Autodesk Inventor part; units mm, degrees
(part 2 of 5)
  arc A560 (53.3588, 33.4823) -> (53.3762, 34.0151) centre (44.1675, 34.0494) ccw
  arc A561 (53.3762, 34.0151) -> (53.35, 34.4073) centre (50.5813, 34.0255) ccw
  arc A562 (53.35, 34.4073) -> (53.2888, 34.6516) centre (52.1975, 34.2484) ccw
  arc A563 (53.2888, 34.6516) -> (53.1912, 34.6976) centre (53.2166, 34.6249) ccw
  arc A564 (53.1912, 34.6976) -> (53.0949, 34.5943) centre (53.2411, 34.5546) ccw
  arc A565 (53.0949, 34.5943) -> (53.0197, 34.2521) centre (56.5471, 33.6564) ccw
  arc A566 (53.0197, 34.2521) -> (52.9689, 33.8102) centre (57.178, 33.5498) ccw
  arc A567 (52.9689, 33.8102) -> (52.9556, 33.3026) centre (60.0929, 33.3695) ccw
  arc A568 (52.9556, 33.3026) -> (52.9918, 32.5531) centre (62.5862, 33.3929) ccw
  arc A569 (52.9918, 32.5531) -> (53.1004, 32.0963) centre (54.5989, 32.6938) ccw
  arc A570 (53.1004, 32.0963) -> (53.3273, 31.7245) centre (54.3072, 32.5775) ccw
  arc A571 (53.3273, 31.7245) -> (53.7593, 31.2868) centre (57.031, 34.9486) ccw
  arc A572 (53.7593, 31.2868) -> (54.451, 30.7656) centre (57.2206, 35.1607) ccw
  arc A573 (54.451, 30.7656) -> (55.1201, 30.4611) centre (55.9058, 33.0742) ccw
  arc A574 (55.1201, 30.4611) -> (55.827, 30.353) centre (55.8555, 32.9072) ccw
  arc A575 (55.827, 30.353) -> (56.6313, 30.4233) centre (55.8729, 34.466) ccw
  arc A576 (56.6313, 30.4233) -> (57.3715, 30.6596) centre (56.0502, 33.5213) ccw
  arc A577 (57.3715, 30.6596) -> (57.9882, 31.0614) centre (56.3036, 32.9725) ccw
  arc A578 (57.9882, 31.0614) -> (58.495, 31.6477) centre (56.0896, 33.2152) ccw
  arc A579 (58.495, 31.6477) -> (58.91, 32.432) centre (54.3994, 34.3166) ccw
  arc A580 (58.91, 32.432) -> (59.1195, 33.0043) centre (52.6519, 35.0468) ccw
  arc A581 (59.1195, 33.0043) -> (59.1777, 33.3919) centre (57.9219, 33.3825) ccw
  arc A582 (59.1777, 33.3919) -> (59.116, 33.7952) centre (57.759, 33.3813) ccw
  arc A583 (59.116, 33.7952) -> (58.895, 34.4396) centre (49.6346, 30.903) ccw
  arc A584 (58.895, 34.4396) -> (58.0584, 35.697) centre (55.6947, 33.2174) ccw
  arc A585 (58.0584, 35.697) -> (56.7897, 36.4169) centre (55.9863, 33.5232) ccw
  arc A586 (56.7897, 36.4169) -> (55.3538, 36.4458) centre (56.0154, 33.6283) ccw
  arc A587 (55.3538, 36.4458) -> (54.0494, 35.7849) centre (56.0619, 33.4305) ccw
  arc A588 (54.8024, 34.5354) -> (54.6127, 34.3248) centre (56.7247, 32.6131) ccw
  arc A589 (54.6127, 34.3248) -> (54.4523, 34.1018) centre (56.4725, 32.8176) ccw
  arc A590 (54.4523, 34.1018) -> (54.3389, 33.8976) centre (56.1058, 33.0507) ccw
  arc A591 (54.3389, 33.8976) -> (54.3067, 33.7556) centre (54.6352, 33.7556) ccw
  arc A592 (54.3067, 33.7556) -> (54.3603, 33.7064) centre (54.356, 33.7556) ccw
  arc A593 (54.3603, 33.7064) -> (54.4852, 33.7476) centre (54.335, 33.9932) ccw
  arc A594 (54.4852, 33.7476) -> (54.6809, 33.895) centre (53.8225, 34.8311) ccw
  arc A595 (54.6809, 33.895) -> (54.9146, 34.1274) centre (51.9402, 36.884) ccw
  arc A596 (55.4388, 34.573) -> (54.9146, 34.1274) centre (57.0426, 32.1552) ccw
  arc A597 (55.9442, 34.7544) -> (55.4388, 34.573) centre (56.06, 33.6365) ccw
  arc A598 (56.4234, 34.6683) -> (55.9442, 34.7544) centre (56.0346, 33.8814) ccw
  arc A599 (56.871, 34.33) -> (56.4234, 34.6683) centre (55.7592, 33.3238) ccw
  arc A600 (57.1706, 33.8594) -> (56.871, 34.33) centre (55.6391, 33.2151) ccw
  arc A601 (57.2614, 33.3581) -> (57.1706, 33.8594) centre (56.0901, 33.4049) ccw
  arc A602 (57.1308, 32.8701) -> (57.2614, 33.3581) centre (56.1135, 33.4039) ccw
  arc A603 (56.7955, 32.4375) -> (57.1308, 32.8701) centre (55.7467, 33.5964) ccw
  arc A604 (56.2855, 32.1688) -> (56.7955, 32.4375) centre (56.0159, 33.2989) ccw
  arc A605 (55.6751, 32.1559) -> (56.2855, 32.1688) centre (55.9506, 33.5728) ccw
  arc A606 (55.1505, 32.3917) -> (55.6751, 32.1559) centre (55.9154, 33.3919) ccw
  arc A607 (54.8713, 32.8115) -> (55.1505, 32.3917) centre (55.6216, 33.0077) ccw
  arc A608 (54.8713, 32.8115) -> (54.8067, 32.997) centre (53.6761, 32.499) ccw
  arc A609 (54.8067, 32.997) -> (54.7175, 33.1537) centre (53.9996, 32.6414) ccw
  arc A610 (54.7175, 33.1537) -> (54.6187, 33.2616) centre (54.2266, 32.8034) ccw
  arc A611 (54.6187, 33.2616) -> (54.5257, 33.296) centre (54.5257, 33.1529) ccw
  arc A612 (54.5257, 33.296) -> (54.3612, 33.2114) centre (54.5257, 33.094) ccw
  arc A613 (54.3612, 33.2114) -> (54.3373, 33.0302) centre (54.5195, 33.0984) ccw
  arc A614 (54.3373, 33.0302) -> (54.5145, 32.7303) centre (55.2706, 33.3793) ccw
  arc A615 (54.5145, 32.7303) -> (54.8804, 32.3477) centre (58.2611, 35.9463) ccw
  arc A616 (54.8804, 32.3477) -> (55.9513, 31.8532) centre (56.1579, 33.7075) ccw
  arc A617 (55.9513, 31.8532) -> (57.0009, 32.1572) centre (56.1093, 33.2717) ccw
  arc A618 (57.0009, 32.1572) -> (57.5221, 33.1113) centre (56.1209, 33.2573) ccw
  arc A619 (57.5221, 33.1113) -> (57.2647, 34.2552) centre (55.6965, 33.3015) ccw
  arc A620 (57.2647, 34.2552) -> (56.7605, 34.7922) centre (55.7376, 33.3265) ccw
  arc A621 (56.7605, 34.7922) -> (56.1131, 35.0368) centre (55.9537, 33.6361) ccw
  arc A622 (56.1131, 35.0368) -> (55.4239, 34.9447) centre (55.9519, 33.62) ccw
  arc A623 (55.4239, 34.9447) -> (54.8024, 34.5354) centre (56.1069, 33.231) ccw
  arc A624 (-8.5753, 18.557) -> (-9.5884, 17.8072) centre (-7.4577, 15.9877) ccw
  arc A625 (-9.5884, 17.8072) -> (-10.2034, 16.6702) centre (-7.2414, 15.803) ccw
  arc A626 (-10.2034, 16.6702) -> (-10.2979, 15.3835) centre (-7.2545, 15.8068) ccw
  arc A627 (-10.2979, 15.3835) -> (-9.8473, 14.2125) centre (-7.5618, 15.764) ccw
  arc A628 (-9.8473, 14.2125) -> (-9.2705, 13.5192) centre (-6.0196, 16.811) ccw
  arc A629 (-9.2705, 13.5192) -> (-8.6427, 13.0645) centre (-7.4741, 15.3382) ccw
  arc A630 (-8.6427, 13.0645) -> (-7.8947, 12.8111) centre (-7.4197, 15.4441) ccw
  arc A631 (-7.8947, 12.8111) -> (-6.9536, 12.7252) centre (-6.9354, 18.1284) ccw
  arc A632 (-6.9536, 12.7252) -> (-6.336, 12.7642) centre (-6.9379, 17.3929) ccw
  arc A633 (-6.336, 12.7642) -> (-5.8924, 12.8936) centre (-6.5295, 14.2527) ccw
  arc A634 (-5.8924, 12.8936) -> (-5.471, 13.1648) centre (-6.6912, 14.5976) ccw
  arc A635 (-5.471, 13.1648) -> (-4.9086, 13.684) centre (-11.6768, 20.4522) ccw
  arc A636 (-4.9086, 13.684) -> (-4.411, 14.224) centre (-11.2514, 20.0268) ccw
  arc A637 (-4.411, 14.224) -> (-4.1325, 14.6456) centre (-6.0238, 15.5922) ccw
  arc A638 (-4.1325, 14.6456) -> (-3.9927, 15.0708) centre (-5.5046, 15.3323) ccw
  arc A639 (-3.9927, 15.0708) -> (-3.9471, 15.6051) centre (-7.0638, 15.6021) ccw
  arc A640 (-3.9471, 15.6051) -> (-4.3362, 17.2016) centre (-7.4313, 15.6017) ccw
  arc A641 (-4.3362, 17.2016) -> (-5.4057, 18.3728) centre (-7.0463, 15.8007) ccw
  arc A642 (-5.4057, 18.3728) -> (-6.9304, 18.858) centre (-7.081, 15.7462) ccw
  arc A643 (-6.9304, 18.858) -> (-8.5753, 18.557) centre (-7.1082, 15.1842) ccw
  arc A644 (-5.0676, 17.5621) -> (-6.0617, 18.3185) centre (-7.0176, 16.0308) ccw
  arc A645 (-4.5149, 16.3843) -> (-5.0676, 17.5621) centre (-7.3415, 15.7764) ccw
  arc A646 (-4.5323, 15.0755) -> (-4.5149, 16.3843) centre (-7.3806, 15.768) ccw
  arc A647 (-5.1236, 13.9563) -> (-4.5323, 15.0755) centre (-7.042, 15.6857) ccw
  arc A648 (-6.1586, 13.2185) -> (-5.1236, 13.9563) centre (-7.3077, 15.9252) ccw
  arc A649 (-7.3762, 13.0161) -> (-6.1586, 13.2185) centre (-7.1869, 15.6406) ccw
  arc A650 (-8.5324, 13.3913) -> (-7.3762, 13.0161) centre (-7.1936, 15.5474) ccw
  arc A651 (-9.3986, 14.2647) -> (-8.5324, 13.3913) centre (-7.132, 15.6467) ccw
  arc A652 (-9.8202, 15.4116) -> (-9.3986, 14.2647) centre (-6.7098, 15.9041) ccw
  arc A653 (-9.7596, 16.6062) -> (-9.8202, 15.4116) centre (-6.9556, 15.8651) ccw
  arc A654 (-9.2308, 17.6322) -> (-9.7596, 16.6062) centre (-7.1749, 15.9231) ccw
  arc A655 (-8.3301, 18.308) -> (-9.2308, 17.6322) centre (-7.3596, 16.0766) ccw
  arc A656 (-7.6602, 18.5637) -> (-8.3301, 18.308) centre (-5.1957, 11.1012) ccw
  arc A657 (-7.2029, 18.6383) -> (-7.6602, 18.5637) centre (-7.196, 17.1583) ccw
  arc A658 (-6.7429, 18.5682) -> (-7.2029, 18.6383) centre (-7.196, 17.1392) ccw
  arc A659 (-6.0617, 18.3185) -> (-6.7429, 18.5682) centre (-9.2143, 10.7734) ccw
  arc A660 (21.9375, 18.6785) -> (21.2521, 18.2462) centre (22.7945, 16.5601) ccw
  arc A661 (21.2521, 18.2462) -> (20.6532, 17.5458) centre (23.7974, 15.4639) ccw
  arc A662 (20.6532, 17.5458) -> (20.2389, 16.716) centre (23.8344, 15.4393) ccw
  arc A663 (20.2389, 16.716) -> (20.0986, 15.9013) centre (22.5332, 15.9013) ccw
  arc A664 (20.0986, 15.9013) -> (20.3331, 14.6091) centre (23.7765, 15.9013) ccw
  arc A665 (20.3331, 14.6091) -> (21.0026, 13.5913) centre (22.9134, 15.5774) ccw
  arc A666 (21.0026, 13.5913) -> (22.0595, 12.9458) centre (22.9898, 15.6568) ccw
  arc A667 (22.0595, 12.9458) -> (23.4037, 12.7216) centre (23.4037, 16.8629) ccw
  arc A668 (23.4037, 12.7216) -> (24.0232, 12.7586) centre (23.4037, 17.9326) ccw
  arc A669 (24.0232, 12.7586) -> (24.4764, 12.8763) centre (23.8167, 14.4837) ccw
  arc A670 (24.4764, 12.8763) -> (24.8908, 13.1137) centre (23.7803, 14.5723) ccw
  arc A671 (24.8908, 13.1137) -> (25.3894, 13.5366) centre (21.1307, 18.0521) ccw
  arc A672 (25.3894, 13.5366) -> (26.0721, 14.3661) centre (22.4584, 16.6443) ccw
  arc A673 (26.0721, 14.3661) -> (26.4259, 15.2474) centre (23.8366, 15.7754) ccw
  arc A674 (26.4259, 15.2474) -> (26.4378, 16.169) centre (24.0135, 15.7394) ccw
  arc A675 (26.4378, 16.169) -> (26.1195, 17.1169) centre (23.112, 15.5796) ccw
  arc A676 (26.1195, 17.1169) -> (25.3823, 18.053) centre (23.3757, 15.7144) ccw
  arc A677 (25.3823, 18.053) -> (24.3198, 18.6802) centre (23.0864, 15.3772) ccw
  arc A678 (24.3198, 18.6802) -> (23.1067, 18.9027) centre (23.0873, 15.3797) ccw
  arc A679 (23.1067, 18.9027) -> (21.9375, 18.6785) centre (23.0898, 15.8302) ccw
  arc A680 (25.0676, 17.907) -> (24.4535, 18.3079) centre (23.6748, 16.4442) ccw
  arc A681 (25.5832, 17.2676) -> (25.0676, 17.907) centre (22.904, 15.6348) ccw
  arc A682 (25.9297, 16.4923) -> (25.5832, 17.2676) centre (22.7225, 15.5242) ccw
  arc A683 (26.0478, 15.6919) -> (25.9297, 16.4923) centre (23.278, 15.6919) ccw
  arc A684 (25.8118, 14.6865) -> (26.0478, 15.6919) centre (23.7893, 15.6919) ccw
  arc A685 (25.1402, 13.7967) -> (25.8118, 14.6865) centre (23.1012, 16.0339) ccw
  arc A686 (24.1642, 13.1834) -> (25.1402, 13.7967) centre (22.948, 16.2021) ccw
  arc A687 (23.0607, 12.9695) -> (24.1642, 13.1834) centre (23.0607, 15.9222) ccw
  arc A688 (22.1837, 13.1907) -> (23.0607, 12.9695) centre (23.0607, 14.8187) ccw
  arc A689 (21.3717, 13.8262) -> (22.1837, 13.1907) centre (23.6298, 15.875) ccw
  arc A690 (20.7947, 14.721) -> (21.3717, 13.8262) centre (23.7847, 16.0156) ccw
  arc A691 (20.5944, 15.6877) -> (20.7947, 14.721) centre (23.0274, 15.6877) ccw
  arc A692 (20.6629, 16.5519) -> (20.5944, 15.6877) centre (26.0747, 15.6877) ccw
  arc A693 (20.8765, 17.1929) -> (20.6629, 16.5519) centre (22.7147, 16.2243) ccw
  arc A694 (21.2753, 17.7094) -> (20.8765, 17.1929) centre (22.5589, 16.3063) ccw
  arc A695 (21.9116, 18.1874) -> (21.2753, 17.7094) centre (24.0571, 14.6687) ccw
  arc A696 (22.5682, 18.5221) -> (21.9116, 18.1874) centre (24.4333, 14.0517) ccw
  arc A697 (23.1084, 18.6436) -> (22.5682, 18.5221) centre (23.1842, 17.0457) ccw
  arc A698 (23.6816, 18.5777) -> (23.1084, 18.6436) centre (23.1931, 16.857) ccw
  arc A699 (24.4535, 18.3079) -> (23.6816, 18.5777) centre (21.8067, 11.9734) ccw
  line L44 (-25.521, 15.4111) -> (-28.7346, 12.1514)
  line L45 (-28.7346, 12.1514) -> (-28.7346, 9.5915)
  arc A700 (-28.7346, 9.5915) -> (-28.6366, 7.4521) centre (-5.3387, 9.5916) ccw
  arc A701 (-28.6366, 7.4521) -> (-28.1931, 6.6742) centre (-27.559, 7.5511) ccw
  arc A702 (-28.1931, 6.6742) -> (-27.2267, 6.3494) centre (-27.1884, 8.0636) ccw
  arc A703 (-27.2267, 6.3494) -> (-24.2411, 6.3421) centre (-25.5497, 81.3851) ccw
  line L46 (-24.2411, 6.3421) -> (-20.8891, 6.4005)
  line L47 (-20.8891, 6.4005) -> (-17.9331, 8.8541)
  arc A704 (-17.9331, 8.8541) -> (-16.7781, 9.8218) centre (-121.2357, 133.3124) ccw
  arc A705 (-16.7781, 9.8218) -> (-15.7544, 10.6993) centre (-83.8441, 89.1079) ccw
  arc A706 (-15.7544, 10.6993) -> (-14.9009, 11.4464) centre (-109.465, 118.6117) ccw
  arc A707 (-14.9009, 11.4464) -> (-14.6672, 11.6902) centre (-16.241, 12.9651) ccw
  arc A708 (-14.6672, 11.6902) -> (-14.3935, 12.3476) centre (-15.6467, 12.4836) ccw
  arc A709 (-14.3935, 12.3476) -> (-14.3503, 13.526) centre (-22.601, 13.2384) ccw
  arc A710 (-14.3503, 13.526) -> (-14.4719, 14.6873) centre (-22.752, 13.2331) ccw
  arc A711 (-14.4719, 14.6873) -> (-14.7911, 15.2463) centre (-15.4093, 14.5227) ccw
  arc A712 (-14.7911, 15.2463) -> (-15.5734, 15.7613) centre (-17.2371, 12.3831) ccw
  arc A713 (-15.5734, 15.7613) -> (-18.4192, 17.1422) centre (-134.5724, -225.8672) ccw
  arc A714 (-18.4192, 17.1422) -> (-21.3756, 18.5416) centre (-205.3974, -374.0441) ccw
  arc A715 (-21.3756, 18.5416) -> (-21.9558, 18.6708) centre (-21.9558, 17.3038) ccw
  arc A716 (-21.9558, 18.6708) -> (-22.1818, 18.5848) centre (-21.9558, 18.3308) ccw
  arc A717 (-22.1818, 18.5848) -> (-23.148, 17.7133) centre (41.8537, -53.3805) ccw
  arc A718 (-23.148, 17.7133) -> (-24.2639, 16.6604) centre (9.8095, -18.3331) ccw
  arc A719 (-24.2639, 16.6604) -> (-25.521, 15.4111) centre (36.2511, -45.4888) ccw
  arc A720 (-20.7472, 17.667) -> (-20.8023, 17.9318) centre (-20.9032, 17.7726) ccw
  arc A721 (-21.2749, 16.9723) -> (-20.7472, 17.667) centre (-27.3541, 22.1388) ccw
  arc A722 (-22.2857, 15.8621) -> (-21.2749, 16.9723) centre (-38.0254, 31.2079) ccw
  arc A723 (-24.2727, 13.8483) -> (-22.2857, 15.8621) centre (-191.8838, 181.2158) ccw
  arc A724 (-25.7552, 12.3729) -> (-24.2727, 13.8483) centre (-261.3043, 250.5361) ccw
  arc A725 (-27.0248, 11.13) -> (-25.7552, 12.3729) centre (-148.8704, 136.8545) ccw
  arc A726 (-28.1562, 10.0351) -> (-27.0248, 11.13) centre (-759.4677, 766.8912) ccw
  arc A727 (-28.2459, 9.9977) -> (-28.1562, 10.0351) centre (-28.2488, 10.1309) ccw
  arc A728 (-28.2953, 10.04) -> (-28.2459, 9.9977) centre (-28.247, 10.0464) ccw
  arc A729 (-28.3217, 10.2959) -> (-28.2953, 10.04) centre (-24.0914, 10.6026) ccw
  arc A730 (-28.3323, 10.6251) -> (-28.3217, 10.2959) centre (-24.2267, 10.5927) ccw
  arc A731 (-28.3198, 11.0167) -> (-28.3323, 10.6251) centre (-20.1629, 10.5607) ccw
  arc A732 (-28.2628, 11.5092) -> (-28.3198, 11.0167) centre (-24.1529, 10.7838) ccw
  arc A733 (-28.1497, 11.889) -> (-28.2628, 11.5092) centre (-26.5581, 11.2083) ccw
  arc A734 (-27.9718, 12.184) -> (-28.1497, 11.889) centre (-27.0029, 11.3985) ccw
  arc A735 (-27.7203, 12.4184) -> (-27.9718, 12.184) centre (-27.0101, 11.4044) ccw
  arc A736 (-27.7203, 12.4184) -> (-26.8678, 13.1252) centre (-31.6394, 18.0136) ccw
  arc A737 (-26.8678, 13.1252) -> (-25.2239, 14.7654) centre (-100.5465, 88.6085) ccw
  arc A738 (-25.2239, 14.7654) -> (-23.4487, 16.586) centre (-360.2394, 343.201) ccw
  arc A739 (-23.4487, 16.586) -> (-23.4502, 16.7741) centre (-23.545, 16.6793) ccw
  arc A740 (-23.4547, 16.8311) -> (-23.4502, 16.7741) centre (-23.419, 16.8053) ccw
  arc A741 (-23.3801, 16.9045) -> (-23.4547, 16.8311) centre (-23.2004, 16.6472) ccw
  arc A742 (-23.2389, 16.9834) -> (-23.3801, 16.9045) centre (-22.9169, 16.2414) ccw
  arc A743 (-23.0484, 17.0548) -> (-23.2389, 16.9834) centre (-22.4455, 15.1552) ccw
  arc A744 (-23.0484, 17.0548) -> (-22.8604, 17.1345) centre (-23.3781, 18.0935) ccw
  arc A745 (-22.8604, 17.1345) -> (-22.7243, 17.2385) centre (-23.1201, 17.6156) ccw
  arc A746 (-22.7243, 17.2385) -> (-22.6597, 17.3487) centre (-22.9263, 17.431) ccw
  arc A747 (-22.6597, 17.3487) -> (-22.6725, 17.4492) centre (-22.7767, 17.3848) ccw
  arc A748 (-22.6931, 17.5364) -> (-22.6725, 17.4492) centre (-22.5521, 17.5237) ccw
  arc A749 (-22.6551, 17.6117) -> (-22.6931, 17.5364) centre (-22.5791, 17.5261) ccw
  arc A750 (-22.557, 17.6626) -> (-22.6551, 17.6117) centre (-22.5053, 17.4431) ccw
  arc A751 (-22.4136, 17.6793) -> (-22.557, 17.6626) centre (-22.4136, 17.0535) ccw
  arc A752 (-22.4136, 17.6793) -> (-22.2711, 17.6974) centre (-22.4136, 18.2493) ccw
  arc A753 (-22.2711, 17.6974) -> (-22.1753, 17.7521) centre (-22.3235, 17.9003) ccw
  arc A754 (-22.1753, 17.7521) -> (-22.1404, 17.8331) centre (-22.2597, 17.8365) ccw
  arc A755 (-22.1404, 17.8331) -> (-22.1657, 17.9272) centre (-22.3101, 17.8379) ccw
  arc A756 (-22.1085, 18.0969) -> (-22.1657, 17.9272) centre (-22.0668, 17.9883) ccw
  arc A757 (-21.7429, 18.1655) -> (-22.1085, 18.0969) centre (-21.7395, 17.1381) ccw
  arc A758 (-21.2237, 18.1076) -> (-21.7429, 18.1655) centre (-21.7352, 15.878) ccw
  arc A759 (-20.8023, 17.9318) -> (-21.2237, 18.1076) centre (-21.5259, 16.7901) ccw
  arc A760 (-25.2569, 10.6462) -> (-23.4654, 12.4279) centre (-410.0261, 399.3194) ccw
  arc A761 (-26.7855, 9.1443) -> (-25.2569, 10.6462) centre (-225.2095, 212.6273) ccw
  arc A762 (-28.1534, 7.8116) -> (-26.7855, 9.1443) centre (-1541.8494, 1562.8338) ccw
  arc A763 (-28.2389, 7.7731) -> (-28.1534, 7.8116) centre (-28.2491, 7.9099) ccw
  arc A764 (-28.2864, 7.8082) -> (-28.2389, 7.7731) centre (-28.2422, 7.8182) ccw
  arc A765 (-28.3197, 7.9951) -> (-28.2864, 7.8082) centre (-26.2641, 8.265) ccw
  arc A766 (-28.3397, 8.2441) -> (-28.3197, 7.9951) centre (-25.8505, 8.3194) ccw
  arc A767 (-28.3398, 8.5417) -> (-28.3397, 8.2441) centre (-23.3628, 8.3945) ccw
  arc A768 (-28.1634, 9.1246) -> (-28.3398, 8.5417) centre (-27.1747, 8.5072) ccw
  arc A769 (-27.583, 9.9256) -> (-28.1634, 9.1246) centre (-22.071, 5.3207) ccw
  arc A770 (-26.4859, 11.147) -> (-27.583, 9.9256) centre (-10.0003, -4.7636) ccw
  arc A771 (-24.2497, 13.4374) -> (-26.4859, 11.147) centre (173.1762, -181.5518) ccw
  arc A772 (-21.6723, 16.027) -> (-24.2497, 13.4374) centre (312.8226, -319.4758) ccw
  arc A773 (-20.6595, 16.9411) -> (-21.6723, 16.027) centre (-11.9773, 6.3028) ccw
  arc A774 (-20.0352, 17.3055) -> (-20.6595, 16.9411) centre (-19.1898, 15.1403) ccw
  arc A775 (-19.4992, 17.3144) -> (-20.0352, 17.3055) centre (-19.7552, 16.5883) ccw
  arc A776 (-19.2978, 17.0004) -> (-19.4992, 17.3144) centre (-19.6002, 17.0281) ccw
  arc A777 (-19.497, 16.5109) -> (-19.2978, 17.0004) centre (-20.202, 17.0831) ccw
  arc A778 (-20.3875, 15.5185) -> (-19.497, 16.5109) centre (-29.9535, 24.9979) ccw
  arc A779 (-23.4654, 12.4279) -> (-20.3875, 15.5185) centre (-643.5197, 633.0134) ccw
  line L48 (-17.0774, 16.1416) -> (-15.8267, 15.5954)
  line L49 (-15.8267, 15.5954) -> (-20.109, 11.3078)
  arc A780 (-20.109, 11.3078) -> (-21.7338, 9.6633) centre (130.6219, -139.2383) ccw
  arc A781 (-21.7338, 9.6633) -> (-23.0607, 8.2797) centre (50.7279, -61.1555) ccw
  arc A782 (-23.0607, 8.2797) -> (-24.1742, 7.0904) centre (210.3258, -211.3379) ccw
  arc A783 (-24.1742, 7.0904) -> (-24.1437, 7.0202) centre (-24.1437, 7.0619) ccw
  arc A784 (-24.1437, 7.0202) -> (-23.9775, 7.086) centre (-24.1437, 7.2631) ccw
  arc A785 (-23.9775, 7.086) -> (-22.7365, 8.256) centre (-290.236, 290.7304) ccw
  arc A786 (-22.7365, 8.256) -> (-21.3271, 9.6145) centre (-99.1095, 88.9043) ccw
  arc A787 (-21.3271, 9.6145) -> (-19.7012, 11.2272) centre (-166.4853, 157.5858) ccw
  arc A788 (-17.7135, 13.1934) -> (-19.7012, 11.2272) centre (123.9383, -131.9961) ccw
  arc A789 (-16.4092, 14.404) -> (-17.7135, 13.1934) centre (7.2039, -12.3463) ccw
  arc A790 (-15.4793, 15.1912) -> (-16.4092, 14.404) centre (3.1328, -7.7344) ccw
  arc A791 (-15.2121, 15.1898) -> (-15.4793, 15.1912) centre (-15.3466, 15.0278) ccw
  arc A792 (-15.0957, 15.0124) -> (-15.2121, 15.1898) centre (-15.4435, 14.911) ccw
  arc A793 (-14.9947, 14.5962) -> (-15.0957, 15.0124) centre (-19.6026, 13.6987) ccw
  arc A794 (-14.9193, 14.0788) -> (-14.9947, 14.5962) centre (-20.3824, 13.5468) ccw
  arc A795 (-14.8854, 13.5121) -> (-14.9193, 14.0788) centre (-22.5082, 13.3398) ccw
  arc A796 (-14.9916, 12.4286) -> (-14.8854, 13.5121) centre (-19.4189, 13.4096) ccw
  arc A797 (-15.3677, 11.644) -> (-14.9916, 12.4286) centre (-16.8626, 12.8432) ccw
  arc A798 (-16.2599, 10.7266) -> (-15.3677, 11.644) centre (-20.6101, 15.8493) ccw
  arc A799 (-18.8728, 8.5413) -> (-16.2599, 10.7266) centre (-162.903, 183.4113) ccw
  line L50 (-18.8728, 8.5413) -> (-21.0334, 6.7617)
  line L51 (-21.0334, 6.7617) -> (-24.5101, 6.7873)
  arc A800 (-25.8512, 6.8107) -> (-24.5101, 6.7873) centre (-24.0218, 73.2143) ccw
  arc A801 (-26.9997, 6.8607) -> (-25.8512, 6.8107) centre (-24.8605, 42.7697) ccw
  arc A802 (-27.9767, 6.9247) -> (-26.9997, 6.8607) centre (-22.1053, 89.0209) ccw
  arc A803 (-28.1032, 7.0013) -> (-27.9767, 6.9247) centre (-27.9651, 7.0867) ccw
  arc A804 (-28.0733, 7.2656) -> (-28.1032, 7.0013) centre (-27.9202, 7.1144) ccw
  arc A805 (-23.4732, 11.9164) -> (-28.0733, 7.2656) centre (3540.804, -3518.0697) ccw
  arc A806 (-18.906, 16.5198) -> (-23.4732, 11.9164) centre (2547.6443, -2534.4612) ccw
  arc A807 (-18.5118, 16.686) -> (-18.906, 16.5198) centre (-18.5064, 16.1226) ccw
  arc A808 (-18.3903, 16.6655) -> (-18.5118, 16.686) centre (-18.5084, 16.3363) ccw
  arc A809 (-18.0147, 16.5268) -> (-18.3903, 16.6655) centre (-25.8175, -4.0316) ccw
  arc A810 (-17.57, 16.3507) -> (-18.0147, 16.5268) centre (-23.9652, 0.8488) ccw
  arc A811 (-17.0774, 16.1416) -> (-17.57, 16.3507) centre (-27.565, -7.877) ccw
  arc A812 (31.4904, 16.7497) -> (29.8015, 15.8256) centre (43.7766, -7.7092) ccw
  arc A813 (29.8015, 15.8256) -> (28.9907, 15.1249) centre (31.3567, 13.2065) ccw
  arc A814 (28.9907, 15.1249) -> (28.6937, 14.382) centre (30.0387, 14.2752) ccw
  arc A815 (28.6937, 14.382) -> (28.786, 13.4143) centre (31.4872, 14.1602) ccw
  arc A816 (28.786, 13.4143) -> (28.9153, 13.0304) centre (32.3143, 14.3886) ccw
  arc A817 (28.9153, 13.0304) -> (29.1033, 12.6062) centre (34.7394, 15.3576) ccw
  arc A818 (29.1033, 12.6062) -> (29.3168, 12.2073) centre (34.5545, 15.2673) ccw
  arc A819 (29.3168, 12.2073) -> (29.5236, 11.9034) centre (31.6223, 13.5542) ccw
  arc A820 (29.5236, 11.9034) -> (29.9117, 11.5437) centre (30.8547, 12.9504) ccw
  arc A821 (29.9117, 11.5437) -> (30.3658, 11.3533) centre (30.6252, 12.608) ccw
  arc A822 (30.3658, 11.3533) -> (31.1221, 11.2591) centre (31.3308, 16.0212) ccw
  arc A823 (31.1221, 11.2591) -> (32.9597, 11.193) centre (36.2486, 128.214) ccw
  arc A824 (34.8458, 11.1153) -> (32.9597, 11.193) centre (30.931, -60.9936) ccw
  arc A825 (35.7892, 10.9839) -> (34.8458, 11.1153) centre (34.5388, 5.4609) ccw
  arc A826 (36.6288, 10.7028) -> (35.7892, 10.9839) centre (34.8139, 6.6759) ccw
  arc A827 (37.9781, 10.0568) -> (36.6288, 10.7028) centre (23.3175, -18.8328) ccw
  arc A828 (37.9781, 10.0568) -> (38.8125, 9.6534) centre (48.8551, 31.4907) ccw
  arc A829 (38.8125, 9.6534) -> (39.6028, 9.3128) centre (46.2807, 25.8927) ccw
  arc A830 (39.6028, 9.3128) -> (40.2738, 9.0585) centre (46.0914, 25.4228) ccw
  arc A831 (40.2738, 9.0585) -> (40.5937, 9.0033) centre (40.5937, 9.9583) ccw
  arc A832 (40.5937, 9.0033) -> (41.0377, 9.0921) centre (40.5937, 10.1575) ccw
  arc A833 (41.0377, 9.0921) -> (41.4567, 9.3492) centre (40.4272, 10.5572) ccw
  arc A834 (41.4567, 9.3492) -> (41.8024, 9.7431) centre (40.2781, 10.7322) ccw
  arc A835 (41.8024, 9.7431) -> (42.0321, 10.2292) centre (40.1159, 10.8374) ccw
  arc A836 (42.0321, 10.2292) -> (42.0456, 10.849) centre (40.9832, 10.5621) ccw
  arc A837 (42.0456, 10.849) -> (41.3292, 13.4175) centre (-113.5207, -31.1607) ccw
  arc A838 (41.3292, 13.4175) -> (40.579, 15.868) centre (-32.0771, -7.7147) ccw
  arc A839 (40.579, 15.868) -> (40.0123, 17.2455) centre (31.3045, 12.8577) ccw
  line L52 (40.0123, 17.2455) -> (39.6688, 17.9272)
  line L53 (39.6688, 17.9272) -> (36.7516, 17.9272)
  line L54 (36.7516, 17.9272) -> (33.8345, 17.9272)
  line L55 (33.8345, 17.9272) -> (31.4904, 16.7497)
  arc A840 (32.6743, 14.9524) -> (31.6334, 13.8961) centre (83.5815, -36.2514) ccw
  arc A841 (31.6334, 13.8961) -> (30.7813, 12.9826) centre (57.9157, -11.4751) ccw
  arc A842 (30.7813, 12.9826) -> (30.0777, 12.1928) centre (98.2555, -47.8357) ccw
  arc A843 (30.0777, 12.1928) -> (30.0814, 12.0758) centre (30.1419, 12.1363) ccw
  arc A844 (30.0814, 12.0758) -> (30.1988, 12.0722) centre (30.142, 12.1363) ccw
  arc A845 (30.1988, 12.0722) -> (31.0249, 12.8123) centre (-38.7867, 89.9127) ccw
  arc A846 (31.0249, 12.8123) -> (31.9787, 13.7047) centre (4.2219, 42.4137) ccw
  arc A847 (31.9787, 13.7047) -> (33.0829, 14.7935) centre (-22.8936, 70.4594) ccw
  line L56 (33.0829, 14.7935) -> (35.9346, 17.6611)
  line L57 (35.9346, 17.6611) -> (37.6194, 17.6482)
  arc A848 (38.2778, 17.6353) -> (37.6194, 17.6482) centre (37.4072, -10.0048) ccw
  arc A849 (38.8613, 17.607) -> (38.2778, 17.6353) centre (37.7375, 0.4809) ccw
  arc A850 (39.3485, 17.5699) -> (38.8613, 17.607) centre (37.315, -5.957) ccw
  arc A851 (39.481, 17.526) -> (39.3485, 17.5699) centre (39.3225, 17.2696) ccw
  arc A852 (39.4959, 17.4256) -> (39.481, 17.526) centre (39.4461, 17.4696) ccw
  arc A853 (38.8083, 16.6552) -> (39.4959, 17.4256) centre (-27.4262, 76.4559) ccw
  arc A854 (37.9713, 15.7589) -> (38.8083, 16.6552) centre (11.7054, 41.1255) ccw
  arc A855 (36.9429, 14.7148) -> (37.9713, 15.7589) centre (-15.291, 67.1977) ccw
  arc A856 (36.9429, 14.7148) -> (35.9022, 13.6667) centre (124.5614, -73.3214) ccw
  arc A857 (35.9022, 13.6667) -> (35.0255, 12.7561) centre (83.6206, -33.1524) ccw
  arc A858 (35.0255, 12.7561) -> (34.2733, 11.9559) centre (193.5492, -137.0039) ccw
  arc A859 (34.2733, 11.9559) -> (34.228, 11.8411) centre (34.3961, 11.8411) ccw
  arc A860 (34.228, 11.8411) -> (34.3505, 11.7795) centre (34.3047, 11.8411) ccw
  arc A861 (34.3505, 11.7795) -> (34.8959, 12.2204) centre (29.2097, 18.6966) ccw
  arc A862 (34.8959, 12.2204) -> (35.7997, 13.0552) centre (18.7939, 30.5594) ccw
  arc A863 (35.7997, 13.0552) -> (37.4152, 14.6395) centre (-132.8, 186.5964) ccw
  arc A864 (38.3095, 15.5198) -> (37.4152, 14.6395) centre (197.3399, -146.9215) ccw
  arc A865 (39.0735, 16.2611) -> (38.3095, 15.5198) centre (121.0585, -69.0041) ccw
  arc A866 (39.7561, 16.9167) -> (39.0735, 16.2611) centre (604.5313, -571.8219) ccw
  arc A867 (39.8032, 16.9356) -> (39.7561, 16.9167) centre (39.8032, 16.8676) ccw
  arc A868 (39.8348, 16.9128) -> (39.8032, 16.9356) centre (39.8032, 16.9023) ccw
  arc A869 (39.889, 16.7393) -> (39.8348, 16.9128) centre (34.8558, 15.2621) ccw
  arc A870 (39.9454, 16.5235) -> (39.889, 16.7393) centre (36.2968, 15.6851) ccw
  arc A871 (39.9993, 16.2674) -> (39.9454, 16.5235) centre (33.0493, 14.9388) ccw
  arc A872 (39.9764, 15.8278) -> (39.9993, 16.2674) centre (39.0937, 16.0942) ccw
  arc A873 (39.7542, 15.3792) -> (39.9764, 15.8278) centre (38.5322, 16.2637) ccw
  arc A874 (39.2395, 14.773) -> (39.7542, 15.3792) centre (35.5882, 18.3947) ccw
  arc A875 (38.1205, 13.6718) -> (39.2395, 14.773) centre (-6.7837, 60.423) ccw
  arc A876 (38.1205, 13.6718) -> (37.3626, 12.9214) centre (62.5319, -11.7436) ccw
  arc A877 (37.3626, 12.9214) -> (36.75, 12.2641) centre (50.1037, 0.4356) ccw
  arc A878 (36.75, 12.2641) -> (36.2676, 11.7056) centre (58.9648, -7.4134) ccw
  arc A879 (36.2676, 11.7056) -> (36.2727, 11.5858) centre (36.3354, 11.6485) ccw
  arc A880 (36.2727, 11.5858) -> (36.3934, 11.5789) centre (36.3369, 11.65) ccw
  arc A881 (36.3934, 11.5789) -> (36.9427, 12.0279) centre (19.8012, 32.4411) ccw
  arc A882 (36.9427, 12.0279) -> (37.591, 12.6017) centre (26.2744, 24.7324) ccw
  arc A883 (37.591, 12.6017) -> (38.3305, 13.3137) centre (15.3334, 36.4605) ccw
  arc A884 (39.0636, 14.0371) -> (38.3305, 13.3137) centre (142.0884, -91.1196) ccw
  arc A885 (39.6925, 14.6462) -> (39.0636, 14.0371) centre (93.0951, -41.1126) ccw
  arc A886 (40.2519, 15.181) -> (39.6925, 14.6462) centre (331.2423, -289.7672) ccw
  arc A887 (40.3004, 15.2004) -> (40.2519, 15.181) centre (40.3004, 15.1301) ccw
  arc A888 (40.3344, 15.1775) -> (40.3004, 15.2004) centre (40.3004, 15.1638) ccw
  arc A889 (40.398, 15.0113) -> (40.3344, 15.1775) centre (35.9351, 13.3994) ccw
  arc A890 (40.4659, 14.8033) -> (40.398, 15.0113) centre (37.0708, 13.8096) ccw
  arc A891 (40.533, 14.5565) -> (40.4659, 14.8033) centre (34.1451, 12.9532) ccw
  arc A892 (40.5474, 14.151) -> (40.533, 14.5565) centre (39.5916, 14.3202) ccw
  arc A893 (40.3962, 13.7655) -> (40.5474, 14.151) centre (39.5136, 14.334) ccw
  arc A894 (40.0092, 13.2777) -> (40.3962, 13.7655) centre (37.7327, 15.4811) ccw
  arc A895 (39.1678, 12.4369) -> (40.0092, 13.2777) centre (14.4162, 38.0484) ccw
  arc A896 (39.1678, 12.4369) -> (38.5946, 11.8589) centre (52.4583, -1.3154) ccw
  arc A897 (38.5946, 11.8589) -> (38.1394, 11.3447) centre (45.6518, 5.1526) ccw
  arc A898 (38.1394, 11.3447) -> (37.8023, 10.9153) centre (47.0346, 4.0129) ccw
  arc A899 (37.8023, 10.9153) -> (37.8112, 10.791) centre (37.8785, 10.8583) ccw
  arc A900 (37.8112, 10.791) -> (37.9343, 10.7815) centre (37.8783, 10.8581) ccw
  arc A901 (37.9343, 10.7815) -> (38.3358, 11.0916) centre (32.3524, 18.4241) ccw
  arc A902 (38.3358, 11.0916) -> (38.8181, 11.5164) centre (32.9438, 17.6993) ccw
  arc A903 (38.8181, 11.5164) -> (39.3582, 12.0534) centre (27.2868, 23.6536) ccw
  arc A904 (39.8904, 12.5975) -> (39.3582, 12.0534) centre (70.5915, -17.961) ccw
  arc A905 (40.348, 13.0439) -> (39.8904, 12.5975) centre (55.2436, -2.6844) ccw
  arc A906 (40.7453, 13.4169) -> (40.348, 13.0439) centre (83.1063, -32.1046) ccw
  arc A907 (40.7945, 13.4137) -> (40.7453, 13.4169) centre (40.7684, 13.3921) ccw
  arc A908 (40.8286, 13.3536) -> (40.7945, 13.4137) centre (40.6391, 13.2857) ccw
  arc A909 (40.9639, 12.9728) -> (40.8286, 13.3536) centre (-32.2114, -12.8214) ccw
  arc A910 (41.1172, 12.5283) -> (40.9639, 12.9728) centre (9.0491, 1.7229) ccw
  arc A911 (41.2877, 12.0146) -> (41.1172, 12.5283) centre (-14.9999, -6.3805) ccw
  arc A912 (41.5056, 11.2852) -> (41.2877, 12.0146) centre (27.106, 7.3799) ccw
  arc A913 (41.5812, 10.8254) -> (41.5056, 11.2852) centre (39.2923, 10.6849) ccw
  arc A914 (41.5475, 10.4644) -> (41.5812, 10.8254) centre (40.4062, 10.7533) ccw
  arc A915 (41.4053, 10.0976) -> (41.5475, 10.4644) centre (39.9773, 10.8619) ccw
  arc A916 (41.2542, 9.8621) -> (41.4053, 10.0976) centre (39.8465, 10.9318) ccw
  arc A917 (41.0617, 9.6425) -> (41.2542, 9.8621) centre (39.5859, 11.1299) ccw
  arc A918 (40.859, 9.4688) -> (41.0617, 9.6425) centre (39.7731, 10.9413) ccw
  arc A919 (40.6791, 9.3771) -> (40.859, 9.4688) centre (40.4922, 9.9661) ccw
  arc A920 (40.4177, 9.3778) -> (40.6791, 9.3771) centre (40.5496, 9.7854) ccw
  arc A921 (39.7711, 9.6059) -> (40.4177, 9.3778) centre (44.4567, 21.8584) ccw
  arc A922 (39.0003, 9.9301) -> (39.7711, 9.6059) centre (44.3222, 21.5066) ccw
  arc A923 (38.1642, 10.3389) -> (39.0003, 9.9301) centre (47.1509, 27.6598) ccw
  arc A924 (38.1642, 10.3389) -> (36.9915, 10.9109) centre (26.0294, -13.0497) ccw
  arc A925 (36.9915, 10.9109) -> (36.0985, 11.2553) centre (33.7274, 3.7762) ccw
  arc A926 (36.0985, 11.2553) -> (35.2307, 11.4666) centre (34.1174, 5.0064) ccw
  arc A927 (35.2307, 11.4666) -> (34.1575, 11.6091) centre (32.8492, -2.3531) ccw
  line L58 (34.1575, 11.6091) -> (32.2556, 11.7873)
  line L59 (32.2556, 11.7873) -> (35.0264, 14.4773)
  arc A928 (35.0264, 14.4773) -> (36.0764, 15.5212) centre (-8.3823, 59.1897) ccw
  arc A929 (36.0764, 15.5212) -> (36.9324, 16.428) centre (13.5949, 37.6032) ccw
  arc A930 (36.9324, 16.428) -> (37.6284, 17.2071) centre (-12.9075, 61.6499) ccw
  arc A931 (37.6284, 17.2071) -> (37.6242, 17.3404) centre (37.5553, 17.2715) ccw
  arc A932 (37.6242, 17.3404) -> (37.4895, 17.3448) centre (37.5545, 17.2707) ccw
  arc A933 (37.4895, 17.3448) -> (36.6251, 16.5768) centre (96.6684, -50.1285) ccw
  arc A934 (36.6251, 16.5768) -> (35.6232, 15.6417) centre (62.0937, -11.7177) ccw
  arc A935 (35.6232, 15.6417) -> (34.4662, 14.4978) centre (87.9415, -38.4335) ccw
  arc A936 (32.4205, 12.4942) -> (34.4662, 14.4978) centre (-31.1671, 79.4632) ccw
  arc A937 (31.3468, 11.6944) -> (32.4205, 12.4942) centre (28.5478, 16.5729) ccw
  arc A938 (30.6098, 11.5578) -> (31.3468, 11.6944) centre (30.7837, 12.6758) ccw
  arc A939 (29.9661, 11.916) -> (30.6098, 11.5578) centre (30.7733, 12.6092) ccw
  arc A940 (29.5171, 12.604) -> (29.9661, 11.916) centre (32.3454, 13.9594) ccw
  arc A941 (29.4774, 13.1614) -> (29.5171, 12.604) centre (30.2034, 12.9329) ccw
  arc A942 (29.8418, 13.8122) -> (29.4774, 13.1614) centre (31.2209, 12.6127) ccw
  arc A943 (30.9405, 15.0113) -> (29.8418, 13.8122) centre (53.6275, -6.8779) ccw
  arc A944 (32.2443, 16.2979) -> (30.9405, 15.0113) centre (57.8114, -10.9146) ccw
  arc A945 (33.2211, 17.0908) -> (32.2443, 16.2979) centre (38.2011, 9.9578) ccw
  arc A946 (34.0262, 17.5318) -> (33.2211, 17.0908) centre (35.6487, 13.6137) ccw
  arc A947 (34.7606, 17.6784) -> (34.0262, 17.5318) centre (34.7633, 15.7518) ccw
  arc A948 (34.9328, 17.5252) -> (34.7606, 17.6784) centre (34.7608, 17.5052) ccw
  arc A949 (34.85, 17.2242) -> (34.9328, 17.5252) centre (34.5196, 17.4771) ccw
  arc A950 (34.2666, 16.5528) -> (34.85, 17.2242) centre (29.1587, 21.58) ccw
  arc A951 (32.6743, 14.9524) -> (34.2666, 16.5528) centre (-113.7798, 162.2604) ccw
  arc A952 (30.121, 14.6502) -> (30.7256, 15.2087) centre (11.6797, 35.2239) ccw
  arc A953 (29.5924, 14.1995) -> (30.121, 14.6502) centre (20.7196, 25.1388) ccw
  arc A954 (29.1436, 13.8442) -> (29.5924, 14.1995) centre (14.4683, 32.8458) ccw
  arc A955 (29.0507, 13.8501) -> (29.1436, 13.8442) centre (29.1005, 13.9) ccw
  arc A956 (29.0172, 13.9354) -> (29.0507, 13.8501) centre (29.1319, 13.9313) ccw
  arc A957 (29.0352, 14.1341) -> (29.0172, 13.9354) centre (30.8459, 13.8692) ccw
  arc A958 (29.0853, 14.3795) -> (29.0352, 14.1341) centre (31.2516, 13.8099) ccw
  arc A959 (29.1673, 14.6475) -> (29.0853, 14.3795) centre (32.477, 13.4877) ccw
  arc A960 (29.5211, 15.1638) -> (29.1673, 14.6475) centre (30.3004, 14.2505) ccw
  arc A961 (30.4487, 15.8812) -> (29.5211, 15.1638) centre (37.444, 5.8779) ccw
  arc A962 (31.4438, 16.5066) -> (30.4487, 15.8812) centre (37.3107, 6.0686) ccw
  arc A963 (32.0766, 16.682) -> (31.4438, 16.5066) centre (32.1156, 15.3114) ccw
  arc A964 (32.101, 16.6305) -> (32.0766, 16.682) centre (32.0774, 16.6508) ccw
  arc A965 (31.7636, 16.2516) -> (32.101, 16.6305) centre (19.0353, 27.9228) ccw
  arc A966 (31.3076, 15.7758) -> (31.7636, 16.2516) centre (20.795, 26.3092) ccw
  arc A967 (30.7256, 15.2087) -> (31.3076, 15.7758) centre (7.2111, 39.92) ccw
  arc A968 (-61.0772, 15.6012) -> (-61.2967, 15.341) centre (-59.6523, 14.1764) ccw
  arc A969 (-61.2967, 15.341) -> (-61.4688, 15.0481) centre (-59.668, 14.1875) ccw
  arc A970 (-61.4688, 15.0481) -> (-61.5724, 14.7671) centre (-60.0028, 14.3475) ccw
  arc A971 (-61.5724, 14.7671) -> (-61.5806, 14.5477) centre (-61.0947, 14.6394) ccw
  arc A972 (-61.5458, 14.3582) -> (-61.5806, 14.5477) centre (-81.3852, 10.8118) ccw
  arc A973 (-61.5134, 14.1715) -> (-61.5458, 14.3582) centre (-80.1206, 11.0379) ccw
  arc A974 (-61.487, 14.0101) -> (-61.5134, 14.1715) centre (-78.2847, 11.3471) ccw
  arc A975 (-61.4744, 13.9168) -> (-61.487, 14.0101) centre (-63.5568, 13.6819) ccw
  arc A976 (-61.4744, 13.9168) -> (-61.3241, 13.5936) centre (-60.9165, 13.9797) ccw
  arc A977 (-61.3241, 13.5936) -> (-60.9389, 13.2793) centre (-59.9125, 14.9306) ccw
  arc A978 (-60.9389, 13.2793) -> (-60.4426, 13.048) centre (-59.7307, 15.2231) ccw
  arc A979 (-60.4426, 13.048) -> (-59.9504, 12.9695) centre (-59.9504, 14.5519) ccw
  arc A980 (-59.9504, 12.9695) -> (-58.9562, 13.2721) centre (-59.9504, 14.754) ccw
  arc A981 (-58.9562, 13.2721) -> (-58.3355, 14.0698) centre (-59.8549, 14.6117) ccw
  arc A982 (-58.3355, 14.0698) -> (-58.3389, 15.028) centre (-59.6656, 14.5442) ccw
  arc A983 (-58.3389, 15.028) -> (-58.9528, 15.7667) centre (-59.6776, 14.5398) ccw
  arc A984 (-58.9528, 15.7667) -> (-59.6105, 16.0866) centre (-61.2576, 11.865) ccw
  arc A985 (-59.6105, 16.0866) -> (-60.1147, 16.1614) centre (-60.026, 15.0218) ccw
  arc A986 (-60.1147, 16.1614) -> (-60.5729, 16.0074) centre (-60.0378, 15.1739) ccw
  arc A987 (-60.5729, 16.0074) -> (-61.0772, 15.6012) centre (-58.9401, 13.4642) ccw
  arc A988 (-58.852, 15.1221) -> (-59.1182, 15.5546) centre (-59.8938, 14.7789) ccw
  arc A989 (-58.7414, 14.5198) -> (-58.852, 15.1221) centre (-60.9888, 14.4183) ccw
  arc A990 (-58.7975, 13.9245) -> (-58.7414, 14.5198) centre (-60.8965, 14.4225) ccw
  arc A991 (-59.0261, 13.5148) -> (-58.7975, 13.9245) centre (-59.6343, 14.123) ccw
  arc A992 (-59.6224, 13.2469) -> (-59.0261, 13.5148) centre (-59.6769, 14.1656) ccw
  arc A993 (-60.3703, 13.3842) -> (-59.6224, 13.2469) centre (-59.7168, 14.8383) ccw
  arc A994 (-60.9824, 13.8569) -> (-60.3703, 13.3842) centre (-59.69, 14.8979) ccw
  arc A995 (-61.2075, 14.4952) -> (-60.9824, 13.8569) centre (-60.1899, 14.4952) ccw
  arc A996 (-61.0898, 14.9296) -> (-61.2075, 14.4952) centre (-60.3471, 14.4952) ccw
  arc A997 (-60.7234, 15.4229) -> (-61.0898, 14.9296) centre (-58.666, 13.512) ccw
  arc A998 (-60.265, 15.8189) -> (-60.7234, 15.4229) centre (-58.7004, 13.5439) ccw
  arc A999 (-59.8619, 15.9441) -> (-60.265, 15.8189) centre (-59.8619, 15.2328) ccw
  arc A1000 (-59.6984, 15.9166) -> (-59.8619, 15.9441) centre (-59.8619, 15.4447) ccw
  arc A1001 (-59.4973, 15.8297) -> (-59.6984, 15.9166) centre (-60.1801, 14.5262) ccw
  arc A1002 (-59.2934, 15.7036) -> (-59.4973, 15.8297) centre (-60.2808, 14.3339) ccw
  arc A1003 (-59.1182, 15.5546) -> (-59.2934, 15.7036) centre (-60.131, 14.5418) ccw
  arc A1004 (-51.2921, 14.4568) -> (-51.2732, 14.3622) centre (-51.0462, 14.4568) ccw
  arc A1005 (-51.2732, 14.3622) -> (-51.2193, 14.2817) centre (-51.0429, 14.4582) ccw
  arc A1006 (-51.2193, 14.2817) -> (-51.1389, 14.2278) centre (-51.0429, 14.4582) ccw
  arc A1007 (-51.1389, 14.2278) -> (-51.0443, 14.2089) centre (-51.0443, 14.4548) ccw
  arc A1008 (-51.0443, 14.2089) -> (-50.9497, 14.2278) centre (-51.0443, 14.4548) ccw
  arc A1009 (-50.9497, 14.2278) -> (-50.8692, 14.2817) centre (-51.0457, 14.4582) ccw
  arc A1010 (-50.8692, 14.2817) -> (-50.8153, 14.3622) centre (-51.0457, 14.4582) ccw
  arc A1011 (-50.8153, 14.3622) -> (-50.7964, 14.4568) centre (-51.0423, 14.4568) ccw
  arc A1012 (-50.7964, 14.4568) -> (-50.8153, 14.5514) centre (-51.0423, 14.4568) ccw
  arc A1013 (-50.8153, 14.5514) -> (-50.8692, 14.6319) centre (-51.0457, 14.4554) ccw
  arc A1014 (-50.8692, 14.6319) -> (-50.9497, 14.6857) centre (-51.0457, 14.4554) ccw
  arc A1015 (-50.9497, 14.6857) -> (-51.0443, 14.7047) centre (-51.0443, 14.4587) ccw
  arc A1016 (-51.0443, 14.7047) -> (-51.1389, 14.6857) centre (-51.0443, 14.4587) ccw
  arc A1017 (-51.1389, 14.6857) -> (-51.2193, 14.6319) centre (-51.0429, 14.4554) ccw
  arc A1018 (-51.2193, 14.6319) -> (-51.2732, 14.5514) centre (-51.0429, 14.4554) ccw
  arc A1019 (-51.2732, 14.5514) -> (-51.2921, 14.4568) centre (-51.0462, 14.4568) ccw
  arc A1020 (-51.2868, 12.3702) -> (-51.1553, 12.2949) centre (-51.0833, 12.5727) ccw
  arc A1021 (-51.1553, 12.2949) -> (-50.9679, 12.2743) centre (-50.9907, 12.9307) ccw
  arc A1022 (-50.9679, 12.2743) -> (-50.7417, 12.3088) centre (-51.002, 13.2572) ccw
  arc A1023 (-50.7417, 12.3088) -> (-50.4946, 12.3977) centre (-51.1896, 13.9404) ccw
  arc A1024 (-50.4946, 12.3977) -> (-50.142, 12.5615) centre (-57.4094, 27.747) ccw
  arc A1025 (-50.142, 12.5615) -> (-50.1337, 12.61) centre (-50.1551, 12.5887) ccw
  arc A1026 (-50.1337, 12.61) -> (-50.2086, 12.6401) centre (-50.2062, 12.5379) ccw
  arc A1027 (-50.2086, 12.6401) -> (-50.7209, 12.6252) centre (-49.0864, -34.456) ccw
  arc A1028 (-50.7209, 12.6252) -> (-51.0343, 12.5998) centre (-50.6026, 9.2163) ccw
  arc A1029 (-51.0343, 12.5998) -> (-51.2351, 12.5431) centre (-50.9449, 11.8988) ccw
  arc A1030 (-51.2351, 12.5431) -> (-51.3082, 12.4629) centre (-51.1792, 12.4188) ccw
  arc A1031 (-51.3082, 12.4629) -> (-51.2868, 12.3702) centre (-51.223, 12.4338) ccw
  arc A1032 (-37.9064, 11.9127) -> (-38.3723, 11.4777) centre (-37.3748, 10.8762) ccw
  arc A1033 (-38.3723, 11.4777) -> (-38.6129, 10.8035) centre (-36.8281, 10.5465) ccw
  arc A1034 (-38.6129, 10.8035) -> (-38.5754, 10.0717) centre (-36.7339, 10.533) ccw
  arc A1035 (-38.5754, 10.0717) -> (-38.2572, 9.4759) centre (-37.2251, 10.4099) ccw
  arc A1036 (-38.2572, 9.4759) -> (-37.4577, 9.0215) centre (-37.1684, 10.4613) ccw
  arc A1037 (-37.4577, 9.0215) -> (-36.4925, 9.0973) centre (-37.1085, 10.7593) ccw
  arc A1038 (-36.4925, 9.0973) -> (-35.7194, 9.6669) centre (-37.0962, 10.7263) ccw
  arc A1039 (-35.7194, 9.6669) -> (-35.4275, 10.5247) centre (-36.8343, 10.5247) ccw
  arc A1040 (-35.4275, 10.5247) -> (-35.6409, 11.3417) centre (-37.0987, 10.5247) ccw
  arc A1041 (-35.6409, 11.3417) -> (-36.2226, 11.9233) centre (-36.9631, 10.6007) ccw
  arc A1042 (-36.2226, 11.9233) -> (-37.0425, 12.1294) centre (-37.0137, 10.5103) ccw
  arc A1043 (-37.0425, 12.1294) -> (-37.9064, 11.9127) centre (-37.0075, 10.1601) ccw
  arc A1044 (-36.2862, 11.6874) -> (-36.3927, 11.7301) centre (-36.3927, 11.5758) ccw
  arc A1045 (-36.1546, 11.5382) -> (-36.2862, 11.6874) centre (-37.0789, 10.856) ccw
  arc A1046 (-36.0228, 11.327) -> (-36.1546, 11.5382) centre (-37.4433, 10.587) ccw
  arc A1047 (-35.9106, 11.0769) -> (-36.0228, 11.327) centre (-38.1038, 10.243) ccw
  arc A1048 (-35.8831, 10.1515) -> (-35.9106, 11.0769) centre (-37.2319, 10.5745) ccw
  arc A1049 (-36.4375, 9.4447) -> (-35.8831, 10.1515) centre (-37.0957, 10.5318) ccw
  arc A1050 (-37.2875, 9.3095) -> (-36.4375, 9.4447) centre (-37.0285, 10.4208) ccw
  arc A1051 (-38.0163, 9.8021) -> (-37.2875, 9.3095) centre (-37.0081, 10.5083) ccw
  arc A1052 (-38.164, 10.0363) -> (-38.0163, 9.8021) centre (-35.6689, 11.4463) ccw
  arc A1053 (-38.2888, 10.2842) -> (-38.164, 10.0363) centre (-35.6422, 11.4614) ccw
  arc A1054 (-38.3766, 10.511) -> (-38.2888, 10.2842) centre (-36.035, 11.2867) ccw
  arc A1055 (-38.4021, 10.6697) -> (-38.3766, 10.511) centre (-37.8975, 10.6697) ccw
  arc A1056 (-38.2702, 11.0715) -> (-38.4021, 10.6697) centre (-37.7243, 10.6697) ccw
  arc A1057 (-37.8538, 11.5202) -> (-38.2702, 11.0715) centre (-36.096, 9.4712) ccw
  arc A1058 (-37.3624, 11.8525) -> (-37.8538, 11.5202) centre (-36.1631, 9.5494) ccw
  arc A1059 (-36.9993, 11.8732) -> (-37.3624, 11.8525) centre (-37.1579, 11.4599) ccw
  arc A1060 (-36.9993, 11.8732) -> (-36.8394, 11.8184) centre (-36.1661, 14.0445) ccw
  arc A1061 (-36.8394, 11.8184) -> (-36.6673, 11.7721) centre (-36.0077, 14.5683) ccw
  arc A1062 (-36.6673, 11.7721) -> (-36.508, 11.7398) centre (-36.0765, 14.2766) ccw
  arc A1063 (-36.508, 11.7398) -> (-36.3927, 11.7301) centre (-36.3927, 12.4181) ccw
  arc A1064 (46.487, 11.6174) -> (46.0742, 11.1503) centre (50.0679, 8.0366) ccw
  arc A1065 (46.0742, 11.1503) -> (45.9158, 10.8004) centre (46.7188, 10.6477) ccw
  arc A1066 (45.9158, 10.8004) -> (45.9415, 10.4334) centre (46.625, 10.6655) ccw
  arc A1067 (45.9415, 10.4334) -> (46.1636, 9.9166) centre (49.3347, 11.5857) ccw
  arc A1068 (46.1636, 9.9166) -> (46.4582, 9.4579) centre (48.9554, 11.3861) ccw
  arc A1069 (46.4582, 9.4579) -> (46.7668, 9.1898) centre (47.2811, 10.0933) ccw
  arc A1070 (46.7668, 9.1898) -> (47.1676, 9.0519) centre (47.3338, 10.1858) ccw
  arc A1071 (47.1676, 9.0519) -> (47.7613, 9.0071) centre (47.7823, 13.2459) ccw
  arc A1072 (47.7613, 9.0071) -> (48.6944, 9.2774) centre (47.7698, 10.7236) ccw
  arc A1073 (48.6944, 9.2774) -> (49.2625, 9.9984) centre (47.9417, 10.4547) ccw
  arc A1074 (49.2625, 9.9984) -> (49.2617, 10.9183) centre (47.9344, 10.4572) ccw
  arc A1075 (49.2617, 10.9183) -> (48.6958, 11.7121) centre (47.624, 10.3494) ccw
  arc A1076 (48.6958, 11.7121) -> (48.0869, 12.0882) centre (46.7384, 9.2236) ccw
  arc A1077 (48.0869, 12.0882) -> (47.5485, 12.1965) centre (47.5977, 11.0491) ccw
  arc A1078 (47.5485, 12.1965) -> (47.0312, 12.0416) centre (47.5956, 11.0977) ccw
  arc A1079 (47.0312, 12.0416) -> (46.487, 11.6174) centre (48.4715, 9.6329) ccw
  arc A1080 (48.8026, 10.9575) -> (48.272, 11.6133) centre (47.3951, 10.3613) ccw
  arc A1081 (48.8747, 10.15) -> (48.8026, 10.9575) centre (47.585, 10.4417) ccw
  arc A1082 (48.4664, 9.5035) -> (48.8747, 10.15) centre (47.7594, 10.4023) ccw
  arc A1083 (47.7377, 9.2512) -> (48.4664, 9.5035) centre (47.7377, 10.4297) ccw
  arc A1084 (47.2824, 9.3593) -> (47.7377, 9.2512) centre (47.7377, 10.2646) ccw
  arc A1085 (46.8281, 9.6765) -> (47.2824, 9.3593) centre (48.1528, 11.0898) ccw
  arc A1086 (46.4894, 10.1022) -> (46.8281, 9.6765) centre (48.1092, 11.0433) ccw
  arc A1087 (46.3744, 10.5291) -> (46.4894, 10.1022) centre (47.224, 10.5291) ccw
  arc A1088 (46.4787, 10.9184) -> (46.3744, 10.5291) centre (47.1531, 10.5291) ccw
  arc A1089 (46.8275, 11.4235) -> (46.4787, 10.9184) centre (49.7713, 9.0174) ccw
  arc A1090 (47.2426, 11.8573) -> (46.8275, 11.4235) centre (49.8067, 8.9884) ccw
  arc A1091 (47.5586, 11.9779) -> (47.2426, 11.8573) centre (47.5586, 11.5037) ccw
  arc A1092 (47.6642, 11.9565) -> (47.5586, 11.9779) centre (47.5586, 11.7076) ccw
  arc A1093 (47.8477, 11.8708) -> (47.6642, 11.9565) centre (46.5592, 9.3504) ccw
  arc A1094 (48.0586, 11.7529) -> (47.8477, 11.8708) centre (46.3778, 8.9953) ccw
  arc A1095 (48.272, 11.6133) -> (48.0586, 11.7529) centre (45.9713, 8.3285) ccw
  arc A1096 (5.6265, 10.4628) -> (4.4532, 10.0687) centre (7.1428, 4.004) ccw
  arc A1097 (4.4532, 10.0687) -> (3.0849, 9.3784) centre (10.6928, -4.0005) ccw
  arc A1098 (3.0849, 9.3784) -> (1.8204, 8.5738) centre (10.5521, -3.7532) ccw
  arc A1099 (1.8204, 8.5738) -> (0.9913, 7.827) centre (4.5835, 4.6731) ccw
  line L60 (0.9913, 7.827) -> (0.245, 6.9769)
  line L61 (0.245, 6.9769) -> (0.3184, 0.4009)
  line L62 (0.3184, 0.4009) -> (0.3918, -6.175)
  line L63 (0.3918, -6.175) -> (1.3679, -7.0185)
  arc A1100 (1.3679, -7.0185) -> (3.1995, -8.2726) centre (7.8491, 0.4823) ccw
  arc A1101 (3.1995, -8.2726) -> (5.299, -9.1165) centre (8.2149, 1.1712) ccw
  arc A1102 (5.299, -9.1165) -> (7.502, -9.4921) centre (8.1427, 0.9164) ccw
  arc A1103 (7.502, -9.4921) -> (9.6392, -9.3629) centre (8.0432, -0.7007) ccw
  arc A1104 (9.6392, -9.3629) -> (11.6323, -8.7817) centre (7.7828, 0.7122) ccw
  arc A1105 (11.6323, -8.7817) -> (13.6298, -7.7757) centre (6.4628, 3.9678) ccw
  arc A1106 (13.6298, -7.7757) -> (15.2038, -6.6331) centre (7.283, 2.6239) ccw
  arc A1107 (15.2038, -6.6331) -> (15.6447, -5.6978) centre (14.3843, -5.6753) ccw
  arc A1108 (15.6447, -5.6978) -> (15.6476, -5.365) centre (-2.7227, -5.3703) ccw
  arc A1109 (15.6476, -5.365) -> (15.6468, -3.5612) centre (-5692.7869, -7.0173) ccw
  arc A1110 (15.6468, -3.5612) -> (15.6447, -1.4602) centre (-2610.5712, -5.1507) ccw
  arc A1111 (15.6447, -1.4602) -> (15.6406, 0.9471) centre (-4509.3027, -7.8189) ccw
  arc A1112 (15.6406, 0.9471) -> (15.5976, 5.6514) centre (-310.074, 0.3163) ccw
  arc A1113 (15.5976, 5.6514) -> (15.3818, 7.1682) centre (9.4516, 5.5508) ccw
  arc A1114 (15.3818, 7.1682) -> (14.7929, 8.1142) centre (13.5052, 6.6564) ccw
  arc A1115 (14.7929, 8.1142) -> (13.4057, 9.1411) centre (8.1623, 0.6077) ccw
  arc A1116 (13.4057, 9.1411) -> (11.5952, 10.0196) centre (8.0906, 0.4911) ccw
  arc A1117 (11.5952, 10.0196) -> (9.6008, 10.5509) centre (7.7209, -0.5139) ccw
  arc A1118 (9.6008, 10.5509) -> (7.5637, 10.7045) centre (7.7586, -0.292) ccw
  arc A1119 (7.5637, 10.7045) -> (5.6265, 10.4628) centre (7.7265, 1.5176) ccw
  arc A1120 (12.3647, 9.3514) -> (11.2931, 9.8332) centre (9.067, 3.4502) ccw
  arc A1121 (13.5686, 8.5978) -> (12.3647, 9.3514) centre (5.3917, -3.1268) ccw
  arc A1122 (14.621, 7.791) -> (13.5686, 8.5978) centre (5.1495, -3.4742) ccw
  arc A1123 (15.0658, 7.2021) -> (14.621, 7.791) centre (13.5558, 6.5241) ccw
  arc A1124 (15.1706, 6.7635) -> (15.0658, 7.2021) centre (13.9623, 6.7066) ccw
  arc A1125 (15.2384, 5.0679) -> (15.1706, 6.7635) centre (-104.7114, 1.1167) ccw
  arc A1126 (15.2828, 2.9644) -> (15.2384, 5.0679) centre (-73.6845, 2.1388) ccw
  arc A1127 (15.2896, 0.4063) -> (15.2828, 2.9644) centre (-177.8085, 1.1725) ccw
  line L64 (15.2896, 0.4063) -> (15.2649, -5.8358)
  line L65 (15.2649, -5.8358) -> (14.5212, -6.6199)
  arc A1128 (14.1326, -6.9754) -> (14.5212, -6.6199) centre (11.8226, -4.0603) ccw
  arc A1129 (13.5591, -7.4034) -> (14.1326, -6.9754) centre (6.4705, 2.6936) ccw
  arc A1130 (12.9142, -7.8292) -> (13.5591, -7.4034) centre (5.7759, 3.6831) ccw
  arc A1131 (12.2902, -8.1861) -> (12.9142, -7.8292) centre (7.568, 0.7929) ccw
  arc A1132 (11.3376, -8.6389) -> (12.2902, -8.1861) centre (6.2245, 3.3476) ccw
  arc A1133 (10.623, -8.8548) -> (11.3376, -8.6389) centre (10.0016, -5.5071) ccw
  arc A1134 (9.7542, -8.9462) -> (10.623, -8.8548) centre (9.6079, -3.3861) ccw
  arc A1135 (8.0762, -8.9683) -> (9.7542, -8.9462) centre (8.0762, 54.8502) ccw
  arc A1136 (6.5011, -8.9458) -> (8.0762, -8.9683) centre (8.0762, 46.146) ccw
  arc A1137 (5.5786, -8.8608) -> (6.5011, -8.9458) centre (6.7104, -1.6244) ccw
  arc A1138 (4.8379, -8.6756) -> (5.5786, -8.8608) centre (6.2356, -4.6601) ccw
  arc A1139 (3.9861, -8.3286) -> (4.8379, -8.6756) centre (7.7532, -0.3001) ccw
  arc A1140 (3.3963, -8.0198) -> (3.9861, -8.3286) centre (7.237, -1.4003) ccw
  arc A1141 (2.7502, -7.6192) -> (3.3963, -8.0198) centre (9.9054, 3.1988) ccw
  arc A1142 (2.1468, -7.194) -> (2.7502, -7.6192) centre (9.6394, 2.7968) ccw
  arc A1143 (1.6932, -6.812) -> (2.1468, -7.194) centre (5.3039, -2.9843) ccw
  line L66 (1.6932, -6.812) -> (0.7636, -5.9352)
  line L67 (0.7636, -5.9352) -> (0.7636, 0.5235)
  line L68 (0.7636, 0.5235) -> (0.7636, 6.9822)
  line L69 (0.7636, 6.9822) -> (1.3628, 7.6943)
  arc A1144 (2.148, 8.4124) -> (1.3628, 7.6943) centre (4.4913, 5.0619) ccw
  arc A1145 (3.336, 9.1423) -> (2.148, 8.4124) centre (8.878, -1.2105) ccw
  arc A1146 (4.6811, 9.7646) -> (3.336, 9.1423) centre (9.3535, -2.0986) ccw
  arc A1147 (5.9692, 10.1602) -> (4.6811, 9.7646) centre (7.8814, 1.6391) ccw
  arc A1148 (7.2074, 10.3304) -> (5.9692, 10.1602) centre (7.5963, 2.9095) ccw